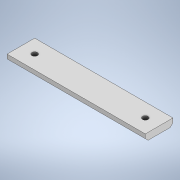
# Autodesk Inventor part: Rail stand
Saved by Autodesk Inventor 2022 (Build 260153000, 153)
## iProperties
Created: 2021-12-04
Part Number: Rail stand
Material: Generic
Document SubType Name: Modeling
Designer: LEGION SMIT
Density: 1 g/cm^3
Appearance: Default
Author: LEGION SMIT
Autodesk Inventor part; units mm, degrees
ref_plane "YZ Plane" through (0, 0, 0) normal (1, 0, 0) x (0, 1, 0)
ref_plane "XZ Plane" through (0, 0, 0) normal (0, 1, 0) x (-1, 0, 0)
ref_plane "XY Plane" through (0, 0, 0) normal (0, 0, 1) x (1, 0, 0)
sketch "Sketch1" plane through (0, 0, 0) normal (0, 1, 0) x (-1, 0, 0)
  line L0 (-50, -10) -> (50, -10)
  line L1 (50, -10) -> (50, 10)
  line L2 (50, 10) -> (-50, 10)
  line L3 (-50, 10) -> (-50, -10)
  line L4 (-50, -10) -> (50, 10) construction
  line L5 (50, -10) -> (-50, 10) construction
  point P0 (0, 0)
  dimension "d0" = 100
  dimension "d1" = 20
  constraints: 12 end point, 2 midpoint, 2 parallel, 1 horizontal, 1 perpendicular
  measures "d0" distance of L2.end L1.end
  measures "d1" distance of L1.end L0.end
extrude "Extrusion1" add sketch "Sketch1" along normal blind 5
sketch "Sketch2" plane through (0, 5, 0) normal (0, 1, 0) x (1, 0, 0)
  line L0 (-50, 10) -> (-50, -10) projected
  line L1 (-50, 0) -> (-40, 0)
  line L2 (50, -10) -> (50, 10) projected
  line L3 (50, 0) -> (40, 0)
  point P0 (0, 0)
  dimension "d4" = 10
  dimension "d5" = 10
  constraints: 4 end point, 2 horizontal, 2 midpoint
  measures "d4" distance of L1.start L1.end
  measures "d5" distance of L3.start L3.end
hole "Hole1" at (-40, 5, 0) direction (0, -1, 0) diameter 4 depth 6
hole "Hole2" at (40, 5, 0) direction (0, -1, 0) diameter 4 depth 6
chamfer "Chamfer1" distance 2 angle 45 2 edges at (0, 0, 10) (0, 0, -10)
thread "Thread1" size "M4x0.7" class "6H" standard "ANSI Metric M Profile" length 5
thread "Thread2" size "M4x0.7" class "6H" standard "ANSI Metric M Profile" length 5
body "Solid1"
